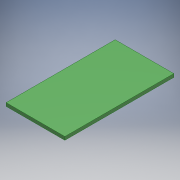
# Autodesk Inventor part: arduino
Saved by Autodesk Inventor 2018 (Build 220112000, 112)
## iProperties
Created: 2017-12-11
Part Number: arduino
Material: Generic
Document SubType Name: Modeling
Designer: caleb
Density: 1 g/cm^3
Appearance: Smooth - Dark Forest Green
Author: caleb
Autodesk Inventor part; units mm, degrees
ref_plane "YZ Plane" through (0, 0, 0) normal (1, 0, 0) x (0, 1, 0)
ref_plane "XZ Plane" through (0, 0, 0) normal (0, 1, 0) x (-1, 0, 0)
ref_plane "XY Plane" through (0, 0, 0) normal (0, 0, 1) x (1, 0, 0)
sketch "Sketch1" plane through (0, 0, 0) normal (0, 0, 1) x (1, 0, 0)
  line L0 (-8.89, -16.51) -> (8.89, -16.51)
  line L1 (8.89, -16.51) -> (8.89, 16.51)
  line L2 (8.89, 16.51) -> (-8.89, 16.51)
  line L3 (-8.89, 16.51) -> (-8.89, -16.51)
  line L4 (-8.89, -16.51) -> (8.89, 16.51) construction
  line L5 (8.89, -16.51) -> (-8.89, 16.51) construction
  point P0 (0, 0)
  point P1 (0, 0)
  point P2 (0, 0)
  dimension "d0" = 33.02
  dimension "d1" = 17.78
  constraints: 12 end point, 3 midpoint, 2 parallel, 1 coincident, 1 horizontal, 1 perpendicular
  measures "d0" distance of L0.end L1.end
  measures "d1" distance of L1.end L2.end
extrude "Extrusion1" add sketch "Sketch1" against normal blind 1
body "Solid1"
